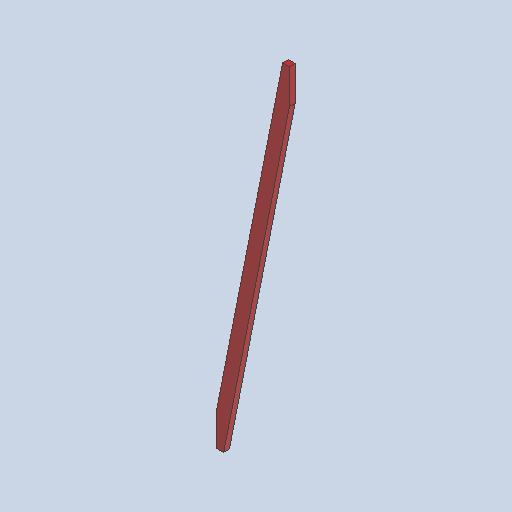
# Autodesk Inventor part: s28x2x4
Saved by Autodesk Inventor 2025.1 (Build 291241020, 241B)
## iProperties
Created: 2024-09-17
Part Number: s28x2x4
Material: Generic
Document SubType Name: Modeling
Designer: User
Density: 1 g/cm^3
Appearance: Default
Stock Number: 10
Author: User
Autodesk Inventor part; units mm, degrees
ref_plane "YZ Plane" through (0, 0, 0) normal (1, 0, 0) x (0, 1, 0)
ref_plane "XZ Plane" through (0, 0, 0) normal (0, 1, 0) x (-1, 0, 0)
ref_plane "XY Plane" through (0, 0, 0) normal (0, 0, 1) x (1, 0, 0)
sketch "Sketch1" plane through (0, 0, 0) normal (0, 0, 1) x (1, 0, 0)
  line L0 (571.5, 0) -> (571.5, 2438.4) projected
  line L1 (88.9, 0) -> (2349.5, 0) projected
  line L2 (88.9, 0) -> (88.9, 2438.4) projected
  line L3 (88.9, 2438.4) -> (2349.5, 2438.4) projected
  line L4 (134.2122, 0) -> (571.5, 2209.4541)
  line L5 (88.9, 228.9459) -> (526.1878, 2438.4)
  line L6 (134.2122, 0) -> (88.9, 0)
  line L7 (526.1878, 2438.4) -> (571.5, 2438.4)
  line L8 (571.5, 2209.4541) -> (571.5, 2438.4)
  line L9 (88.9, 228.9459) -> (88.9, 0)
  point P0 (0, 0)
  constraints: 12 end point, 4 point on line, 3 collinear, 1 parallel, 1 perpendicular, 2 other
extrude "Extrusion1" add sketch "Sketch1" against normal blind 38.1 contours L4 L1 L2 L5 L3 L0
body "Solid1"
